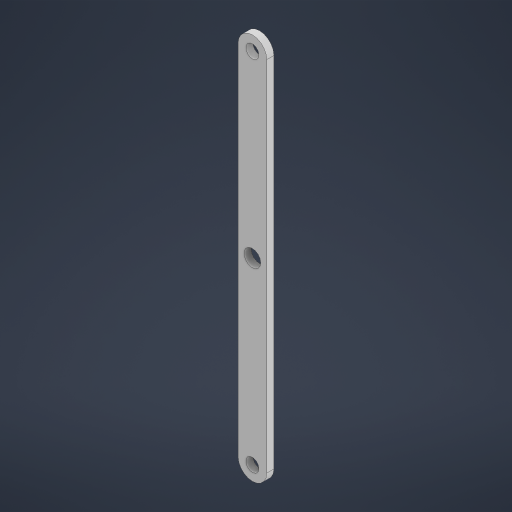
# Autodesk Inventor part: FP V2 Spring Beam
Saved by Autodesk Inventor 2023.6 (Build 276521000, 521)
## iProperties
Created: 2026-02-23
Part Number: FP V2 Spring Beam
Material: Generic
Document SubType Name: Modeling
Designer: user
Density: 1 g/cm^3
Appearance: Default
Author: user
Autodesk Inventor part; units mm, degrees
ref_plane "YZ Plane" through (0, 0, 0) normal (1, 0, 0) x (0, 1, 0)
ref_plane "XZ Plane" through (0, 0, 0) normal (0, 1, 0) x (-1, 0, 0)
ref_plane "XY Plane" through (0, 0, 0) normal (0, 0, 1) x (1, 0, 0)
sketch "Sketch1" plane through (0, 0, 0) normal (0, 0, 1) x (1, 0, 0)
  line L0 (6, -75) -> (-6, -75)
  line L1 (-6, -75) -> (-6, 75)
  line L2 (-6, 75) -> (6, 75)
  line L3 (6, 75) -> (6, -75)
  line L4 (6, -75) -> (-6, 75) construction
  line L5 (-6, -75) -> (6, 75) construction
  circle A0 centre (0, 75) radius 6
  circle A1 centre (0, -75) radius 6
  circle A2 centre (0, -75) radius 2.75
  circle A3 centre (0, 75) radius 2.75
  point P0 (0, 0)
  point P1 (-6, 75)
  dimension "d0" = 12
  dimension "d1" = 150
  dimension "d2" = 5.5
  dimension "d3" = 5.5
  constraints: 12 end point, 4 midpoint, 2 centre point, 2 coincident, 2 parallel, 1 horizontal, 1 perpendicular, 6 other
  measures "d0" distance between parallel lines of L3 L1
  measures "d1" distance between parallel lines of L0 L2
  measures "d2" diameter of A2
  measures "d3" diameter of A3
extrude "Extrusion1" add sketch "Sketch1" along normal blind 3 contours A1 L0 A2 | A1 L1 A0 L3 | L0 A2 A1 | A0 L2 A3 | L2 A3 A0
sketch "Sketch2" plane through (0, 0, 3) normal (0, 0, 1) x (1, 0, 0)
  circle A0 centre (0, 0) radius 3.5
  dimension "d6" = 7
  constraints: 1 centre point, 1 coincident
  measures "d6" diameter of A0
extrude "Extrusion2" cut sketch "Sketch2" against normal blind 5
body "Solid1"
